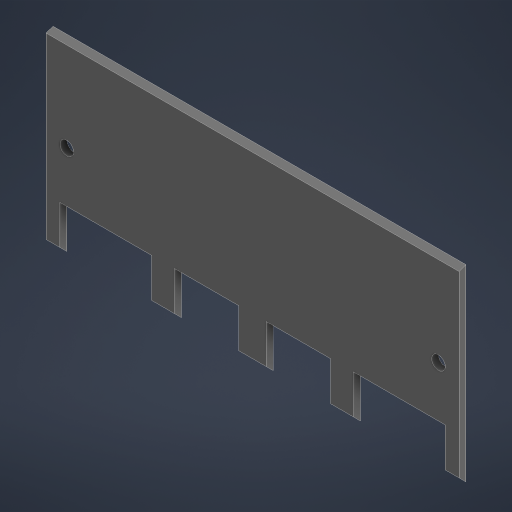
# Autodesk Inventor part: pług_część2
Saved by Autodesk Inventor 2023.4 (Build 274418000, 418)
## iProperties
Created: 2025-10-31
Part Number: pług_część2
Material: Stal
Document SubType Name: Modeling
Designer: Jakub Borsukiewicz
Density: 7.85 g/cm^3
Appearance: Szara
Author: Jakub Borsukiewicz
Autodesk Inventor part; units mm, degrees
ref_plane "YZ Plane" through (0, 0, 0) normal (1, 0, 0) x (0, 1, 0)
ref_plane "XZ Plane" through (0, 0, 0) normal (0, 1, 0) x (-1, 0, 0)
ref_plane "XY Plane" through (0, 0, 0) normal (0, 0, 1) x (1, 0, 0)
sketch "Szkic1" plane through (0, 0, 0) normal (0, 0, 1) x (1, 0, 0)
  line L0 (-63, 0) -> (63, 0) projected
  line L1 (0, -28.7) -> (0, 28.7) projected
  line L2 (-45, -20.5) -> (45, -20.5)
  line L3 (45, -20.5) -> (45, 20.5)
  line L4 (45, 20.5) -> (-45, 20.5)
  line L5 (-45, 20.5) -> (-45, -20.5)
  line L6 (-45, -20.5) -> (45, 20.5) construction
  line L7 (45, -20.5) -> (-45, 20.5) construction
  point P0 (0, 0)
  dimension "d0" = 90
  dimension "d1" = 41
  constraints: 12 end point, 2 midpoint, 2 parallel, 1 horizontal, 1 perpendicular
  measures "d0" distance of L3.end L4.end
  measures "d1" distance of L2.end L3.end
extrude "Wyciągnięcie proste1" add sketch "Szkic1" along normal blind 1.5
sketch "Szkic2" plane through (45, -20.5, 0) normal (1, 0, 0) x (0, 0, -1)
  line L0 (0, 0) -> (0, 41) projected
  line L1 (0, 41) -> (-1.5, 41) projected
  line L2 (-1.5, 0) -> (-1.5, 41) projected
  line L3 (0, 0) -> (-1.5, 0) projected
  line L4 (0, 0) -> (-1.5, 0) projected
  line L5 (0, 0) -> (-1.5, 1.5)
  line L6 (-1.5, 0) -> (-1.5, 41) projected
  line L7 (0, 41) -> (-1.5, 41) projected
  line L8 (0, 41) -> (-1.5, 40.454)
  point P0 (0, 20.5)
  dimension "d4" = 45
  dimension "d5" = 70
  constraints: 4 end point, 2 point on line
  measures "d4" angle of L0 L5
  measures "d5" angle of L0 L8
extrude "Wyciągnięcie proste2" cut sketch "Szkic2" against normal blind 90 contours L3 L2 L5 | L8 L2 L1
sketch "Szkic3" plane through (0, 0, 0) normal (0, 0, -1) x (-1, 0, 0)
  line L0 (45, 20.5) -> (45, -20.5) projected
  line L1 (-45, 20.5) -> (45, 20.5) projected
  point P0 (0, 0)
  point P1 (40.5, 0.5)
  dimension "d8" = 4.5
  dimension "d9" = 20
  measures "d8" distance from line of L0 point (40.5, 0.5)
  measures "d9" distance from line of L1 point (40.5, 0.5)
hole "Otwór1" at (-40.5, 0.5, 0) direction (0, 0, 1) diameter 3 depth 4
sketch "Szkic4" plane through (0, 0, 1.5) normal (0, 0, 1) x (1, 0, 0)
  circle A0 centre (-40.5, 0.5) radius 1.5 projected
  line L0 (-45, -19) -> (45, -19) projected
  line L1 (45, -19) -> (45, 19.954) projected
  line L2 (45, 19.954) -> (-45, 19.954) projected
  line L3 (-45, 19.954) -> (-45, -19) projected
  line L4 (0, -28.7) -> (0, 28.7) projected
  line L5 (-63, 0) -> (63, 0) projected
  line L6 (-45, -20.5) -> (45, -20.5) projected
  line L7 (-45, -20.5) -> (-45, -19) projected
  line L8 (45, -19) -> (45, -20.5) projected
  line L9 (-3, -20.5) -> (-17, -20.5)
  line L10 (-17, -20.5) -> (-17, -10.5)
  line L11 (-17, -10.5) -> (-3, -10.5)
  line L12 (-3, -10.5) -> (-3, -20.5)
  line L13 (-22, -20.5) -> (-42, -20.5)
  line L14 (-42, -20.5) -> (-42, -10.5)
  line L15 (-42, -10.5) -> (-22, -10.5)
  line L16 (-22, -10.5) -> (-22, -20.5)
  point P0 (0, 0)
  point P1 (-42, -20.5)
  dimension "d17" = 14
  dimension "d18" = 20
  dimension "d19" = 10
  dimension "d20" = 10
  dimension "d21" = 5
  dimension "d22" = 3
  constraints: 16 end point, 4 parallel, 2 horizontal, 2 perpendicular, 2 point on line
  measures "d17" distance of L10.end L11.end
  measures "d18" distance of L14.end L15.end
  measures "d19" distance of L13.end L14.end
  measures "d20" distance of L9.end L10.end
  measures "d21" distance between parallel lines of L16 L10
  measures "d22" distance between parallel lines of L4 L12
extrude "Wyciągnięcie proste3" cut sketch "Szkic4" against normal blind 5 contours L14 L15 L16 L0 | L0 L16 L6 L14 | L12 L6 L10 L0 | L0 L10 L11 L12
mirror "Odbij2" about plane through (0, 0, 0) normal (1, 0, 0) of "Wyciągnięcie proste3", "Otwór1"
